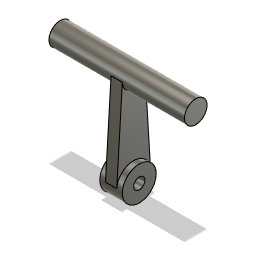
tusk v2 (Autodesk Fusion 360 design; units mm, degrees)
Autodesk Fusion 360 part; units mm, degrees
sketch "Sketch1" plane through (0, 0, 0) normal (1, 0, 0) x (0, 0, -1)
  circle A0 centre (0, 0) radius 2.5
  circle A1 centre (0, 0) radius 7.5
  line L0 (0, 0) -> (0, 40)
  circle A2 centre (0, 40) radius 5
  line L1 (-5, 40) -> (-7.4852, 0.4706)
  line L2 (5, 40) -> (7.4852, 0.4706)
  dimension "d1" = 5
  dimension "d2" = 5
  dimension "d3" = 40
  dimension "d4" = 10
  dimension "d5" = 39.5294
  dimension "d6" = 39.5294
  constraint coincident A0.centre A1.centre
  constraint vertical L0
  constraint coincident L0.end A2.centre
  constraint coincident A2 L1.start
  constraint coincident A1 L1.end
  constraint tangent A1 L1
  constraint coincident A2 L2.start
  constraint coincident A1 L2.end
  constraint tangent A1 L2
  measures "d1" diameter of A0
  measures "d2" distance of A0
  measures "d3" distance of A0.centre L0.end
  measures "d4" diameter of A2
  measures "d5" vertical distance of L2.start L2.end
  measures "d6" vertical distance of L1.start L1.end
extrude "Extrude1" add sketch "Sketch1" along normal mid plane 10 contours A1
extrude "Extrude2" add sketch "Sketch1" along normal mid plane 5 contours A1 L0 A2 L2 | A1 L0 A2 L1
extrude "Extrude3" add sketch "Sketch1" along normal mid plane 60 contours A2
